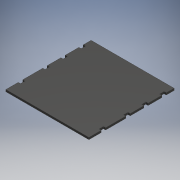
# Autodesk Inventor part: BA09
Saved by Autodesk Inventor 2017 (Build 210142000, 142)
## iProperties
Created: 2019-05-29
Part Number: BA09
Material: Wood (Cherry)
Document SubType Name: Modeling
Designer: Dell
Density: 0.63 g/cm^3
Appearance: Smooth - Black
Author: Dell
Autodesk Inventor part; units mm, degrees
ref_plane "YZ Plane" through (0, 0, 0) normal (1, 0, 0) x (0, 1, 0)
ref_plane "XZ Plane" through (0, 0, 0) normal (0, 1, 0) x (-1, 0, 0)
ref_plane "XY Plane" through (0, 0, 0) normal (0, 0, 1) x (1, 0, 0)
sketch "Sketch1" plane through (0, 0, 0) normal (0, 0, 1) x (1, 0, 0)
  line L0 (0, 0) -> (525.78, 0)
  line L1 (525.78, 0) -> (525.78, 355.6)
  line L2 (525.78, 355.6) -> (0, 355.6)
  line L3 (0, 355.6) -> (0, 0)
  dimension "d0" = 525.78
  dimension "d1" = 355.6
  constraints: 8 end point, 2 parallel, 1 horizontal, 1 perpendicular
  measures "d0" distance of L2.end L1.end
  measures "d1" distance of L2.end L0.start
extrude "Extrusion1" add sketch "Sketch1" along normal blind 12.7
sketch "Sketch2" plane through (0, 0, 12.7) normal (0, 0, 1) x (1, 0, 0)
  line L0 (525.78, 0) -> (525.78, 355.6) projected
  line L1 (525.78, 306.07) -> (511.81, 306.07)
  line L2 (511.81, 306.07) -> (511.81, 278.13)
  line L3 (511.81, 278.13) -> (525.78, 278.13)
  line L4 (525.78, 278.13) -> (525.78, 306.07)
  line L5 (525.78, 191.135) -> (511.81, 191.135)
  line L6 (511.81, 191.135) -> (511.81, 164.465)
  line L7 (511.81, 164.465) -> (525.78, 164.465)
  line L8 (525.78, 164.465) -> (525.78, 191.135)
  line L9 (525.78, 77.47) -> (511.81, 77.47)
  line L10 (511.81, 77.47) -> (511.81, 49.53)
  line L11 (511.81, 49.53) -> (525.78, 49.53)
  line L12 (525.78, 49.53) -> (525.78, 77.47)
  line L13 (0, 306.07) -> (13.97, 306.07)
  line L14 (13.97, 306.07) -> (13.97, 278.13)
  line L15 (13.97, 278.13) -> (0, 278.13)
  line L16 (0, 278.13) -> (0, 306.07)
  line L17 (0, 355.6) -> (0, 0) projected
  line L18 (0, 164.465) -> (13.97, 164.465)
  line L19 (13.97, 164.465) -> (13.97, 191.135)
  line L20 (13.97, 191.135) -> (0, 191.135)
  line L21 (0, 191.135) -> (0, 164.465)
  line L22 (0, 77.47) -> (13.97, 77.47)
  line L23 (13.97, 77.47) -> (13.97, 49.53)
  line L24 (13.97, 49.53) -> (0, 49.53)
  line L25 (0, 49.53) -> (0, 77.47)
  point P0 (0, 177.8)
  point P1 (525.78, 177.8)
  dimension "d4" = 13.97
  dimension "d5" = 13.97
  dimension "d6" = 27.94
  dimension "d7" = 26.67
  dimension "d8" = 27.94
  dimension "d9" = 49.53
  dimension "d10" = 49.53
  constraints: 48 end point, 12 parallel, 8 point on line, 6 horizontal, 6 perpendicular, 5 horizontal alignment, 4 midpoint, 4 vertical alignment
  measures "d4" distance of L13.start L13.end
  measures "d5" distance of L1.start L1.end
  measures "d6" distance of L13.end L14.end
  measures "d7" distance of L18.end L19.end
  measures "d8" distance of L22.end L23.end
  measures "d9" distance of L17.start L13.start
  measures "d10" distance of L17.end L24.end
extrude "Extrusion2" cut sketch "Sketch2" against normal through all
sketch "Sketch3" plane through (0, 0, 12.7) normal (0, 0, 1) x (1, 0, 0)
  line L0 (0, 0) -> (525.78, 0)
  line L1 (525.78, 0) -> (525.78, -184.15)
  line L2 (525.78, -184.15) -> (0, -184.15)
  line L3 (0, -184.15) -> (0, 0)
  line L4 (525.78, 355.6) -> (0, 355.6) projected
  line L5 (0, -78.105) -> (13.97, -78.105)
  line L6 (13.97, -78.105) -> (13.97, -106.045)
  line L7 (13.97, -106.045) -> (0, -106.045)
  line L8 (0, -106.045) -> (0, -78.105)
  line L9 (525.78, -78.105) -> (511.81, -78.105)
  line L10 (511.81, -78.105) -> (511.81, -106.045)
  line L11 (511.81, -106.045) -> (525.78, -106.045)
  line L12 (525.78, -106.045) -> (525.78, -78.105)
  point P0 (525.78, -92.075)
  point P1 (0, -92.075)
  point P2 (13.97, 49.53)
  point P3 (511.81, 49.53)
  dimension "d13" = 539.75
  dimension "d16" = 27.94
  dimension "d17" = 27.94
  constraints: 24 end point, 6 parallel, 4 midpoint, 3 horizontal, 3 perpendicular, 2 point on line, 2 vertical alignment, 1 coincident
  measures "d13" distance between parallel lines of L4 L2
  measures "d16" distance of L5.end L6.end
  measures "d17" distance of L9.end L10.end
extrude "Extrusion3" add sketch "Sketch3" against normal blind 12.7 contours L0 L1 L9 L10 L11 L2 L3 L7 L6 L5
body "Solid1"
